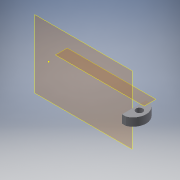
# Autodesk Inventor part: spacer
Saved by Autodesk Inventor 2016 (Build 200138000, 138)
## iProperties
Created: 2016-06-13
Part Number: spacer
Material: Generic
Document SubType Name: Modeling
Designer: ajar021
Density: 1 g/cm^3
Appearance: Default
Author: ajar021
Autodesk Inventor part; units mm, degrees
ref_plane "YZ Plane" through (0, 0, 0) normal (1, 0, 0) x (0, 1, 0)
ref_plane "Work Plane1" through (0, 0, 0) normal (0, 0, 1) x (1, 0, 0)
ref_plane "Work Plane2" through (-2.9544, 5, 3) normal (0, 0, 1) x (1, 0, 0)
ref_plane "Work Plane3" through (-3.1588, -5, 4) normal (0, 0, 1) x (1, 0, 0)
sketch "Sketch4" plane through (0, 0, 0) normal (0, 0, 1) x (1, 0, 0)
  point P0 (0, 0)
ref_plane "Work Plane4" through (4.2892, 3.6962, 0) normal (0, 1, 0) x (1, 0, 0)
sketch "Sketch5" plane through (4.2892, 3.6962, 0) normal (0, 1, 0) x (1, 0, 0)
  line L0 (30.0115, 2.0361) -> (30.0115, -6.9639)
  line L1 (30.0115, -6.9639) -> (31.5115, -6.9639)
  line L2 (31.5115, -6.9639) -> (31.5115, 2.0361) construction
  line L3 (31.5115, 2.0361) -> (30.0115, 2.0361)
  line L4 (31.5115, -2.4639) -> (34.5115, -2.4639) construction
  arc A0 (31.5115, -6.9639) -> (31.5115, 2.0361) centre (29.6365, -2.4639) ccw
  line L5 (31.5115, -2.4639) -> (32.0115, -2.4639)
  circle A1 centre (32.0115, -2.4639) radius 1.25
  point P0 (-4.2892, 0)
  dimension "d10" = 9
  dimension "d11" = 1.5
  dimension "d12" = 0.5
  dimension "d13" = 2.5
  constraints: 12 end point, 3 perpendicular, 3 point on circle, 2 centre point, 1 coincident, 1 horizontal, 1 midpoint, 1 point on line, 1 vertical
  measures "d10" distance of L0.start L0.end
  measures "d11" distance of L0.end L1.end
  measures "d12" distance of L4.start L5.end
  measures "d13" diameter of A1
extrude "Extrusion4" add sketch "Sketch5" against normal blind 3
body "Solid2"
